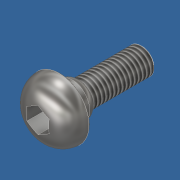
# Autodesk Inventor part: Axel-Male
Saved by Autodesk Inventor 2018 (Build 220112000, 112)
## iProperties
Created: 2018-02-28
Part Number: Axel-Male
Material: Stainless Steel
Document SubType Name: Modeling
Designer: 232963
Density: 8 g/cm^3
Appearance: Semi-Polished
Mass: 8.3022 g
Surface Area: 7.9849 cm^2
Volume: 1.03778 cm^3
Author: 232963
Autodesk Inventor part; units mm, degrees
ref_plane "YZ Plane" through (0, 0, 0) normal (1, 0, 0) x (0, 1, 0)
ref_plane "XZ Plane" through (0, 0, 0) normal (0, 1, 0) x (-1, 0, 0)
ref_plane "XY Plane" through (0, 0, 0) normal (0, 0, 1) x (1, 0, 0)
sketch "Sketch1" plane through (0, 0, 0) normal (0, 0, 1) x (1, 0, 0)
  circle A0 centre (0, 0) radius 6.7056
  dimension "d0" = 13.4112
  constraints: 1 centre point, 1 coincident
  measures "d0" diameter of A0
extrude "Extrusion1" add sketch "Sketch1" along normal blind 5.08
fillet "Fillet1" radius 4.7625 1 edges at (-6.7056, 0, 5.08)
fillet "Fillet2" radius 0.3175 1 edges at (-6.7056, 0, 0)
sketch "Sketch2" plane through (0, 0, 5.08) normal (0, 0, 1) x (1, 0, 0)
  line L0 (0, -2.8575) -> (-2.4747, -1.4288)
  line L1 (-2.4747, -1.4288) -> (-2.4747, 1.4287)
  line L2 (-2.4747, 1.4287) -> (0, 2.8575)
  line L3 (0, 2.8575) -> (2.4747, 1.4287)
  line L4 (2.4747, 1.4287) -> (2.4747, -1.4288)
  line L5 (2.4747, -1.4288) -> (0, -2.8575)
  point P0 (0, 0)
  point P1 (0, 0)
  dimension "d5" = 5.715
  constraints: 12 end point, 1 coincident, 13 other
  measures "d5" distance of L0.start L2.end
extrude "Extrusion2" cut sketch "Sketch2" against normal blind 3.81
sketch "Sketch3" plane through (0, 0, 0) normal (1, 0, 0) x (0, 1, 0)
  line L0 (0, 0) -> (0, -18.288)
  line L1 (0, -18.288) -> (2.921, -18.288)
  line L2 (2.921, -18.288) -> (2.921, -4.318)
  line L3 (2.921, -4.318) -> (3.9497, -4.318)
  line L4 (3.9497, -4.318) -> (3.9497, 0)
  line L5 (6.3881, 0) -> (-6.3881, 0) projected
  dimension "d8" = 2.921
  dimension "d9" = 13.97
  dimension "d10" = 18.288
  dimension "d11" = 3.9497
  constraints: 10 end point, 4 perpendicular, 1 point on line, 1 vertical
  measures "d8" distance of L0.end L1.end
  measures "d9" distance of L1.end L2.end
  measures "d10" distance of L0.start L0.end
  measures "d11" distance between parallel lines of L0 L4
revolve "Revolution1" add sketch "Sketch3" angle 360 about axis through (0, 0, 0) along (0, 0, -1)
fillet "Fillet3" radius 1.905 1 edges at (0, -3.9497, -4.318)
fillet "Fillet4" radius 0.3175 1 edges at (0, -3.9497, 0)
thread "Thread1" size "1/4-28 UNF" class "2A" standard "ANSI Unified Screw Threads" full length
chamfer "Chamfer1" distance 0.3175 angle 45 1 edges at (0, -2.921, -18.288)
body "Solid1"
